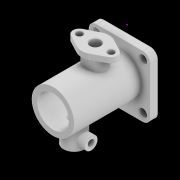
# Autodesk Inventor part: 零件1
Saved by Autodesk Inventor 2020 (Build 240168000, 168)
## iProperties
Created: 2020-11-12
Part Number: 零件1
Material: 常规
Document SubType Name: Modeling
Designer: NH55
Density: 1 g/cm^3
Appearance: 默认
Author: NH55
Autodesk Inventor part; units mm, degrees
sketch "草图1" plane through (0, 0, 0) normal (0, 0, 1) x (1, 0, 0)
  line L0 (22, 29) -> (-22, 29)
  arc A0 (-22, 29) -> (-29, 22) centre (-22, 22) ccw
  line L1 (-29, 22) -> (-29, -22)
  arc A1 (-29, -22) -> (-22, -29) centre (-22, -22) ccw
  line L2 (-22, -29) -> (22, -29)
  arc A2 (22, -29) -> (29, -22) centre (22, -22) ccw
  line L3 (29, -22) -> (29, 22)
  arc A3 (29, 22) -> (22, 29) centre (22, 22) ccw
  circle A4 centre (-22, 22) radius 4
  circle A5 centre (22, 22) radius 4
  circle A6 centre (22, -22) radius 4
  circle A7 centre (-22, -22) radius 4
  point P0 (0, 0)
  point P1 (0, 29)
  point P2 (-29, 0)
  dimension "d0" = 58
  dimension "d1" = 58
  dimension "d2" = 7
  dimension "d3" = 8
  constraints: 8 centre point, 8 end point, 8 point on circle, 8 tangent, 6 equal radius, 4 coincident, 3 perpendicular, 2 midpoint, 1 horizontal, 1 horizontal alignment, 1 vertical alignment
  measures "d0" distance between parallel lines of L3 L1
  measures "d1" distance between parallel lines of L2 L0
  measures "d2" radius of A2
  measures "d3" diameter of A4
extrude "拉伸1" add sketch "草图1" along normal blind 7
sketch "草图2" plane through (0, 0, 0) normal (0, 0, -1) x (-1, 0, 0)
  circle A0 centre (0, 0) radius 20
  dimension "d6" = 40
  constraints: 1 centre point, 1 coincident
  measures "d6" diameter of A0
extrude "拉伸2" add sketch "草图2" against normal blind 70
sketch "草图3" plane through (0, 0, 70) normal (0, 0, 1) x (1, 0, 0)
  circle A0 centre (0, 0) radius 15
  dimension "d9" = 30
  constraints: 1 centre point, 1 coincident
  measures "d9" diameter of A0
extrude "拉伸3" cut sketch "草图3" against normal blind 70
ref_plane "工作平面4" through (0, -36, 0) normal (0, 1, 0) x (-1, 0, 0)
sketch "草图6" plane through (0, -36, 0) normal (0, 1, 0) x (-1, 0, 0)
  line L0 (22, 0) -> (-22, 0) projected
  line L1 (-22, 0) -> (-22, 7) projected
  line L2 (22, 7) -> (-22, 7) projected
  line L3 (22, 0) -> (22, 7) projected
  line L4 (20, 70) -> (-20, 70) projected
  line L5 (-20, 7) -> (20, 7) projected
  circle A0 centre (0, 50) radius 10
  point P0 (0, 0)
  point P1 (0, 70)
  dimension "d16" = 20
  dimension "d17" = 50
  constraints: 1 centre point, 1 midpoint, 1 vertical alignment
  measures "d16" diameter of A0
  measures "d17" distance from line of L0 A0.centre
extrude "拉伸4" add sketch "草图6" along normal up to surface contours A0
sketch "草图7" plane through (0, -36, 50) normal (0, -1, 0) x (1, 0, 0)
  circle A0 centre (0, 0) radius 10 projected
  circle A1 centre (0, 0) radius 5
  point P0 (0, -50)
  dimension "d20" = 10
  constraints: 1 centre point, 1 coincident
  measures "d20" diameter of A1
extrude "拉伸5" cut sketch "草图7" against normal up to surface contours A1
ref_plane "工作平面9" through (0, 36, 30) normal (0, 1, 0) x (1, 0, 0)
sketch "草图9" plane through (0, 36, 30) normal (0, 1, 0) x (1, 0, 0)
  circle A0 centre (0, 0) radius 10
  point P0 (0, 30)
  dimension "d28" = 20
  constraints: 1 centre point
  measures "d28" diameter of A0
extrude "拉伸7" add sketch "草图9" against normal up to surface
ref_plane "工作平面10" through (0, 36, 30) normal (0, 1, 0) x (1, 0, 0)
sketch "草图10" plane through (0, 36, 30) normal (0, 1, 0) x (1, 0, 0)
  circle A0 centre (0, 0) radius 5
  point P0 (0, 30)
  dimension "d31" = 10
  constraints: 1 centre point
  measures "d31" diameter of A0
extrude "拉伸8" cut sketch "草图10" against normal up to surface
sketch "草图11" plane through (0, 36, 30) normal (0, 1, 0) x (1, 0, 0)
  point P0 (0, 30)
sketch "草图12" plane through (0, 36, 30) normal (0, 1, 0) x (1, 0, 0)
  circle A0 centre (0, 0) radius 5 projected
  circle A1 centre (0, 0) radius 10 projected
  line L0 (6.0667, -11.4976) -> (17.8, -5.3066)
  arc A2 (17.8, -5.3066) -> (17.8, 5.3066) centre (15, 0) ccw
  line L1 (17.8, 5.3066) -> (6.0667, 11.4976)
  line L2 (-6.0667, 11.4976) -> (-17.8, 5.3066)
  arc A3 (-17.8, 5.3066) -> (-17.8, -5.3066) centre (-15, 0) ccw
  line L3 (-17.8, -5.3066) -> (-6.0667, -11.4976)
  circle A4 centre (15, 0) radius 3
  arc A5 (6.0667, 11.4976) -> (-6.0667, 11.4976) centre (0, 0) ccw
  arc A6 (-6.0667, -11.4976) -> (6.0667, -11.4976) centre (0, 0) ccw
  circle A7 centre (-15, 0) radius 3
  point P0 (0, 30)
  point P1 (0, -13)
  point P2 (0, 13)
  dimension "d34" = 6
  dimension "d35" = 6
  dimension "d36" = 30
  dimension "d37" = 13
  constraints: 10 point on circle, 8 end point, 8 tangent, 6 centre point, 3 coincident, 3 horizontal alignment, 2 equal radius, 2 vertical alignment, 1 parallel
  measures "d34" radius of A2
  measures "d35" diameter of A4
  measures "d36" distance of A3.centre A2.centre
  measures "d37" radius of A6
extrude "拉伸9" add sketch "草图12" against normal blind 5 contours A6 L3 A3 L2 A5 L1 A2 L0
ref_plane "工作平面11" through (16, 0, 0) normal (1, 0, 0) x (0, 1, 0)
sketch "草图13" plane through (16, 0, 0) normal (1, 0, 0) x (0, 1, 0)
  line L0 (-36, 60) -> (-20, 60) projected
  line L1 (-36, 40) -> (-20, 40) projected
  circle A0 centre (-28, 50) radius 6
  line L2 (0, 84) -> (0, -14) projected
  line L3 (-22, 0) -> (22, 0) projected
  point P0 (0, 0)
  dimension "d41" = 12
  dimension "d42" = 28
  dimension "d43" = 50
  constraints: 1 centre point
  measures "d41" diameter of A0
  measures "d42" distance from line of L2 A0.centre
  measures "d43" distance from line of A0.centre L3
extrude "拉伸10" add sketch "草图13" against normal up to surface
mirror "镜像1" about plane through (0, 0, 0) normal (1, 0, 0) of "拉伸10"
sketch "草图14" plane through (16, -28, 50) normal (1, 0, 0) x (0, 0, -1)
  circle A0 centre (0, 0) radius 3
  point P0 (50, 28)
  dimension "d46" = 6
  constraints: 1 centre point
  measures "d46" diameter of A0
extrude "拉伸11" cut sketch "草图14" against normal up to surface (32 mm away)
